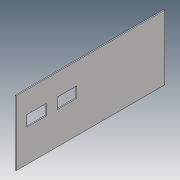
# Autodesk Inventor part: Wall
Saved by Autodesk Inventor 2018.3 (Build 223284000, 284)
## iProperties
Created: 2019-11-07
Part Number: Wall
Material: Generic
Document SubType Name: Modeling
Designer: MattBussey
Density: 1 g/cm^3
Appearance: Default
Author: MattBussey
Autodesk Inventor part; units mm, degrees
ref_plane "YZ Plane" through (0, 0, 0) normal (1, 0, 0) x (0, 1, 0)
ref_plane "XZ Plane" through (0, 0, 0) normal (0, 1, 0) x (-1, 0, 0)
ref_plane "XY Plane" through (0, 0, 0) normal (0, 0, 1) x (1, 0, 0)
sketch "Sketch1" plane through (0, 0, 0) normal (1, 0, 0) x (0, 1, 0)
  line L0 (0, 0) -> (3048, 0)
  line L1 (3048, 0) -> (3048, 7010.4)
  line L2 (3048, 7010.4) -> (0, 7010.4)
  line L3 (0, 7010.4) -> (0, 0)
  line L4 (2032, 6502.4) -> (1524, 6502.4)
  line L5 (1524, 6502.4) -> (1524, 5588)
  line L6 (1524, 5588) -> (2032, 5588)
  line L7 (2032, 5588) -> (2032, 6502.4)
  line L8 (2032, 5080) -> (1524, 5080)
  line L9 (1524, 5080) -> (1524, 4165.6)
  line L10 (1524, 4165.6) -> (2032, 4165.6)
  line L11 (2032, 4165.6) -> (2032, 5080)
  dimension "Width" = 7010.4
  dimension "Height" = 3048
  dimension "d4" = 508
  dimension "d5" = 914.4
  dimension "d6" = 1524
  dimension "d7" = 508
  dimension "d8" = 508
  constraints: 24 end point, 6 parallel, 3 horizontal, 3 perpendicular, 2 point on line, 1 collinear
  measures "Width" distance of L0.end L1.end
  measures "Height" distance of L1.end L2.end
  measures "d4" distance of L4.start L4.end
  measures "d5" distance of L6.end L4.start
  measures "d6" distance between parallel lines of L5 L3
  measures "d7" distance between parallel lines of L2 L4
  measures "d8" distance between parallel lines of L8 L6
extrude "Extrusion1" add sketch "Sketch1" along normal blind 50.8
body "Solid1"
